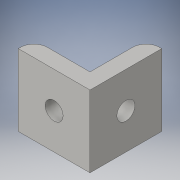
# Autodesk Inventor part: rope connection to cart
Saved by Autodesk Inventor 2016 SP2 (Build 200236200, 236)
## iProperties
Created: 2018-02-01
Part Number: rope connection to cart
Material: Generic
Document SubType Name: Modeling
Designer: CAD
Density: 1 g/cm^3
Appearance: Default
Author: CAD
Autodesk Inventor part; units mm, degrees
ref_plane "YZ Plane" through (0, 0, 0) normal (1, 0, 0) x (0, 1, 0)
ref_plane "XZ Plane" through (0, 0, 0) normal (0, 1, 0) x (-1, 0, 0)
ref_plane "XY Plane" through (0, 0, 0) normal (0, 0, 1) x (1, 0, 0)
sketch "Sketch1" plane through (0, 0, 0) normal (0, 1, 0) x (-1, 0, 0)
  point P0 (0, 0)
sketch "Sketch2" plane through (0, 0, 0) normal (0, 1, 0) x (-1, 0, 0)
  line L0 (-16.4647, 13.2032) -> (-10.9085, 13.2032)
  line L1 (-10.9085, 7.647) -> (-10.9085, -12.1968)
  line L2 (-10.9085, -12.1968) -> (-16.4647, -12.1968)
  line L3 (-16.4647, -12.1968) -> (-16.4647, 13.2032)
  line L4 (-16.4647, 13.2032) -> (8.9353, 13.2032)
  line L5 (8.9353, 13.2032) -> (8.9353, 7.647)
  line L6 (8.9353, 7.647) -> (-10.9085, 7.647)
  line L7 (-16.4647, 7.647) -> (-16.4647, 13.2032)
  point P0 (0, 0)
  dimension "d0" = 5.5563
  dimension "d1" = 25.4
  dimension "d3" = 25.4
  dimension "d4" = 5.5563
  constraints: 16 end point, 4 parallel, 2 horizontal, 2 perpendicular
  measures "d0" distance of L1.end L2.end
  measures "d1" distance of L0.end L1.end
  measures "d3" distance of L0.start L4.end
  measures "d4" distance between parallel lines of L6 L4
extrude "Extrusion1" add sketch "Sketch2" along normal blind 25.4
sketch "Sketch3" plane through (16.4647, 0, 13.2032) normal (1, 0, 0) x (0, 0, -1)
  line L0 (0, 0) -> (25.4, 0) projected
  line L1 (25.4, 0) -> (25.4, 25.4) projected
  point P0 (13.2032, 0)
  point P1 (12.7, 12.7)
  dimension "d7" = 12.7
  dimension "d8" = 12.7
  measures "d7" distance from line of L0 point (12.7, 12.7)
  measures "d8" distance from line of L1 point (12.7, 12.7)
sketch "Sketch4" plane through (-8.9353, 0, 13.2032) normal (0, 0, 1) x (1, 0, 0)
  line L0 (25.4, 0) -> (25.4, 25.4) projected
  line L1 (0, 0) -> (25.4, 0) projected
  point P0 (8.9353, 0)
  point P1 (12.7, 12.7)
  dimension "d9" = 12.7
  dimension "d10" = 12.7
  measures "d9" distance from line of L0 point (12.7, 12.7)
  measures "d10" distance from line of point (12.7, 12.7) L1
hole "Hole1" at (3.7647, 12.7, 13.2032) direction (0, 0, -1) diameter 6.35 end through all
hole "Hole2" at (16.4647, 12.7, 0.5032) direction (-1, 0, 0) diameter 6.35 end through all
fillet "Fillet1" radius 4.7625 2 edges at (10.9085, 12.7, -12.1968) (-8.9353, 12.7, 7.647)
body "Solid1"
